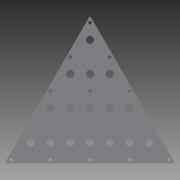
# Autodesk Inventor part: grid16-mask
Saved by Autodesk Inventor 2013 (Build 170138000, 138)
## iProperties
Created: 2013-03-05
Part Number: grid16-mask
Material: Generic
Document SubType Name: Modeling
Designer: Beth Scott
Density: 1 g/cm^3
Author: Beth Scott
Autodesk Inventor part; units mm, degrees
ref_plane "YZ Plane" through (0, 0, 0) normal (1, 0, 0) x (0, 1, 0)
ref_plane "XZ Plane" through (0, 0, 0) normal (0, 1, 0) x (-1, 0, 0)
ref_plane "XY Plane" through (0, 0, 0) normal (0, 0, 1) x (1, 0, 0)
sketch "Triangle 1mm" plane through (0, 0, 0) normal (0, 0, 1) x (1, 0, 0)
  line L0 (0, 0) -> (16.6665, 28.8672) construction
  line L1 (16.6665, 28.8672) -> (33.333, 0) construction
  line L2 (33.333, 0) -> (0, 0) construction
  line L3 (33.333, 0) -> (8.3332, 14.4336) construction
  line L4 (0, 0) -> (24.9997, 14.4336) construction
  line L5 (16.6665, 28.8672) -> (16.6665, 0) construction
  line L6 (0, 14.4336) -> (33.333, 14.4336) construction
  line L7 (0, 19.4336) -> (33.333, 19.4336) construction
  line L8 (0, 9.4336) -> (33.333, 9.4336) construction
  line L9 (16.6665, 19.4336) -> (16.6665, 14.4336) construction
  line L10 (16.6665, 14.4336) -> (16.6665, 9.4336) construction
  circle A0 centre (16.6665, 14.4336) radius 3.5
  point P0 (16.9666, 9.7956)
  dimension "d14" = 33.333
  dimension "d31" = 10
  dimension "d43" = 7
  measures "d14" distance of L1.end L0.start
  measures "d31" distance of L8.start L7.start
  measures "d43" diameter of A0
sketch "Tri16 1mm" plane through (0, 0, 0) normal (0, 0, 1) x (1, 0, 0)
  line L0 (0, 0) -> (16.6665, 28.8672) construction
  line L1 (16.6665, 28.8672) -> (33.333, 0) construction
  line L2 (33.333, 0) -> (0, 0) construction
  line L3 (33.333, 0) -> (8.3333, 14.4336) construction
  line L4 (0, 0) -> (24.9998, 14.4336) construction
  line L5 (16.6665, 28.8672) -> (16.6665, 0) construction
  line L6 (0, 14.4336) -> (33.333, 14.4336) construction
  line L7 (0, 19.4336) -> (33.333, 19.4336) construction
  line L8 (0, 9.4336) -> (33.333, 9.4336) construction
  line L9 (16.6665, 19.4336) -> (16.6665, 14.4336) construction
  line L10 (16.6665, 14.4336) -> (16.6665, 9.4336) construction
  circle A0 centre (16.6665, 14.4336) radius 3.5
  line L11 (33.333, 0) -> (49.9995, 28.8672) construction
  line L12 (49.9995, 28.8672) -> (66.666, 0) construction
  line L13 (66.666, 0) -> (33.333, 0) construction
  line L14 (66.666, 0) -> (41.6663, 14.4336) construction
  line L15 (33.333, 0) -> (58.3328, 14.4336) construction
  line L16 (49.9995, 28.8672) -> (49.9995, 0) construction
  line L17 (33.333, 14.4336) -> (66.666, 14.4336) construction
  line L18 (33.333, 19.4336) -> (66.666, 19.4336) construction
  line L19 (33.333, 9.4336) -> (66.666, 9.4336) construction
  line L20 (49.9995, 19.4336) -> (49.9995, 14.4336) construction
  line L21 (49.9995, 14.4336) -> (49.9995, 9.4336) construction
  circle A1 centre (49.9995, 14.4336) radius 3.5
  line L22 (49.9995, 28.8672) -> (33.333, 0) construction
  line L23 (33.333, 0) -> (16.6665, 28.8672) construction
  line L24 (16.6665, 28.8672) -> (49.9995, 28.8672) construction
  line L25 (16.6665, 28.8672) -> (41.6663, 14.4336) construction
  line L26 (49.9995, 28.8672) -> (24.9998, 14.4336) construction
  line L27 (33.333, 0) -> (33.333, 28.8672) construction
  line L28 (49.9995, 14.4336) -> (16.6665, 14.4336) construction
  line L29 (49.9995, 9.4336) -> (16.6665, 9.4336) construction
  line L30 (49.9995, 19.4336) -> (16.6665, 19.4336) construction
  line L31 (33.333, 9.4336) -> (33.333, 14.4336) construction
  line L32 (33.333, 14.4336) -> (33.333, 19.4336) construction
  circle A2 centre (33.333, 14.4336) radius 3.5
  line L33 (83.3325, 28.8672) -> (66.666, 0) construction
  line L34 (66.666, 0) -> (49.9995, 28.8672) construction
  line L35 (49.9995, 28.8672) -> (83.3325, 28.8672) construction
  line L36 (49.9995, 28.8672) -> (74.9993, 14.4336) construction
  line L37 (83.3325, 28.8672) -> (58.3328, 14.4336) construction
  line L38 (66.666, 0) -> (66.666, 28.8672) construction
  line L39 (83.3325, 14.4336) -> (49.9995, 14.4336) construction
  line L40 (83.3325, 9.4336) -> (49.9995, 9.4336) construction
  line L41 (83.3325, 19.4336) -> (49.9995, 19.4336) construction
  line L42 (66.666, 9.4336) -> (66.666, 14.4336) construction
  line L43 (66.666, 14.4336) -> (66.666, 19.4336) construction
  circle A3 centre (66.666, 14.4336) radius 3.5
  line L44 (66.666, 0) -> (83.3325, 28.8672) construction
  line L45 (83.3325, 28.8672) -> (99.999, 0) construction
  line L46 (99.999, 0) -> (66.666, 0) construction
  line L47 (99.999, 0) -> (74.9993, 14.4336) construction
  line L48 (66.666, 0) -> (91.6658, 14.4336) construction
  line L49 (83.3325, 28.8672) -> (83.3325, 0) construction
  line L50 (66.666, 14.4336) -> (99.999, 14.4336) construction
  line L51 (66.666, 19.4336) -> (99.999, 19.4336) construction
  line L52 (66.666, 9.4336) -> (99.999, 9.4336) construction
  line L53 (83.3325, 19.4336) -> (83.3325, 14.4336) construction
  line L54 (83.3325, 14.4336) -> (83.3325, 9.4336) construction
  circle A4 centre (83.3325, 14.4336) radius 3.5
  line L55 (99.999, 0) -> (116.6655, 28.8672) construction
  line L56 (116.6655, 28.8672) -> (133.332, 0) construction
  line L57 (133.332, 0) -> (99.999, 0) construction
  line L58 (133.332, 0) -> (108.3323, 14.4336) construction
  line L59 (99.999, 0) -> (124.9988, 14.4336) construction
  line L60 (116.6655, 28.8672) -> (116.6655, 0) construction
  line L61 (99.999, 14.4336) -> (133.332, 14.4336) construction
  line L62 (99.999, 19.4336) -> (133.332, 19.4336) construction
  line L63 (99.999, 9.4336) -> (133.332, 9.4336) construction
  line L64 (116.6655, 19.4336) -> (116.6655, 14.4336) construction
  line L65 (116.6655, 14.4336) -> (116.6655, 9.4336) construction
  circle A5 centre (116.6655, 14.4336) radius 3.5
  line L66 (116.6655, 28.8672) -> (99.999, 0) construction
  line L67 (99.999, 0) -> (83.3325, 28.8672) construction
  line L68 (83.3325, 28.8672) -> (116.6655, 28.8672) construction
  line L69 (83.3325, 28.8672) -> (108.3323, 14.4336) construction
  line L70 (116.6655, 28.8672) -> (91.6658, 14.4336) construction
  line L71 (99.999, 0) -> (99.999, 28.8672) construction
  line L72 (116.6655, 14.4336) -> (83.3325, 14.4336) construction
  line L73 (116.6655, 9.4336) -> (83.3325, 9.4336) construction
  line L74 (116.6655, 19.4336) -> (83.3325, 19.4336) construction
  line L75 (99.999, 9.4336) -> (99.999, 14.4336) construction
  line L76 (99.999, 14.4336) -> (99.999, 19.4336) construction
  circle A6 centre (99.999, 14.4336) radius 3.5
  line L77 (16.6665, 28.8672) -> (33.333, 57.7344) construction
  line L78 (33.333, 57.7344) -> (49.9995, 28.8672) construction
  line L79 (49.9995, 28.8672) -> (16.6665, 28.8672) construction
  line L80 (49.9995, 28.8672) -> (24.9998, 43.3008) construction
  line L81 (16.6665, 28.8672) -> (41.6663, 43.3008) construction
  line L82 (33.333, 57.7344) -> (33.333, 28.8672) construction
  line L83 (16.6665, 43.3008) -> (49.9995, 43.3008) construction
  line L84 (16.6665, 48.3008) -> (49.9995, 48.3008) construction
  line L85 (16.6665, 38.3008) -> (49.9995, 38.3008) construction
  line L86 (33.333, 48.3008) -> (33.333, 43.3008) construction
  line L87 (33.333, 43.3008) -> (33.333, 38.3008) construction
  circle A7 centre (33.333, 43.3008) radius 3.5
  line L88 (33.333, 57.7344) -> (49.9995, 86.6017) construction
  line L89 (49.9995, 86.6017) -> (66.666, 57.7344) construction
  line L90 (66.666, 57.7344) -> (33.333, 57.7344) construction
  line L91 (66.666, 57.7344) -> (41.6663, 72.1681) construction
  line L92 (33.333, 57.7344) -> (58.3328, 72.1681) construction
  line L93 (49.9995, 86.6017) -> (49.9995, 57.7344) construction
  line L94 (33.333, 72.1681) -> (66.666, 72.1681) construction
  line L95 (33.333, 77.1681) -> (66.666, 77.1681) construction
  line L96 (33.333, 67.1681) -> (66.666, 67.1681) construction
  line L97 (49.9995, 77.1681) -> (49.9995, 72.1681) construction
  line L98 (49.9995, 72.1681) -> (49.9995, 67.1681) construction
  circle A8 centre (49.9995, 72.1681) radius 3.5
  line L99 (49.9995, 86.6017) -> (66.666, 115.4689) construction
  line L100 (66.666, 115.4689) -> (83.3325, 86.6017) construction
  line L101 (83.3325, 86.6017) -> (49.9995, 86.6017) construction
  line L102 (83.3325, 86.6017) -> (58.3328, 101.0353) construction
  line L103 (49.9995, 86.6017) -> (74.9993, 101.0353) construction
  line L104 (66.666, 115.4689) -> (66.666, 86.6017) construction
  line L105 (49.9995, 101.0353) -> (83.3325, 101.0353) construction
  line L106 (49.9995, 106.0353) -> (83.3325, 106.0353) construction
  line L107 (49.9995, 96.0353) -> (83.3325, 96.0353) construction
  line L108 (66.666, 106.0353) -> (66.666, 101.0353) construction
  line L109 (66.666, 101.0353) -> (66.666, 96.0353) construction
  circle A9 centre (66.666, 101.0353) radius 3.5
  line L110 (66.666, 57.7344) -> (49.9995, 28.8672) construction
  line L111 (49.9995, 28.8672) -> (33.333, 57.7344) construction
  line L112 (33.333, 57.7344) -> (66.666, 57.7344) construction
  line L113 (33.333, 57.7344) -> (58.3328, 43.3008) construction
  line L114 (66.666, 57.7344) -> (41.6663, 43.3008) construction
  line L115 (49.9995, 28.8672) -> (49.9995, 57.7344) construction
  line L116 (66.666, 43.3008) -> (33.333, 43.3008) construction
  line L117 (66.666, 38.3008) -> (33.333, 38.3008) construction
  line L118 (66.666, 48.3008) -> (33.333, 48.3008) construction
  line L119 (49.9995, 38.3008) -> (49.9995, 43.3008) construction
  line L120 (49.9995, 43.3008) -> (49.9995, 48.3008) construction
  circle A10 centre (49.9995, 43.3008) radius 3.5
  line L121 (83.3325, 86.6017) -> (66.666, 57.7344) construction
  line L122 (66.666, 57.7344) -> (49.9995, 86.6017) construction
  line L123 (49.9995, 86.6017) -> (83.3325, 86.6017) construction
  line L124 (49.9995, 86.6017) -> (74.9993, 72.1681) construction
  line L125 (83.3325, 86.6017) -> (58.3328, 72.1681) construction
  line L126 (66.666, 57.7344) -> (66.666, 86.6017) construction
  line L127 (83.3325, 72.1681) -> (49.9995, 72.1681) construction
  line L128 (83.3325, 67.1681) -> (49.9995, 67.1681) construction
  line L129 (83.3325, 77.1681) -> (49.9995, 77.1681) construction
  line L130 (66.666, 67.1681) -> (66.666, 72.1681) construction
  line L131 (66.666, 72.1681) -> (66.666, 77.1681) construction
  circle A11 centre (66.666, 72.1681) radius 3.5
  line L132 (66.666, 57.7344) -> (83.3325, 86.6017) construction
  line L133 (83.3325, 86.6017) -> (99.999, 57.7344) construction
  line L134 (99.999, 57.7344) -> (66.666, 57.7344) construction
  line L135 (99.999, 57.7344) -> (74.9993, 72.1681) construction
  line L136 (66.666, 57.7344) -> (91.6658, 72.1681) construction
  line L137 (83.3325, 86.6017) -> (83.3325, 57.7344) construction
  line L138 (66.666, 72.1681) -> (99.999, 72.1681) construction
  line L139 (66.666, 77.1681) -> (99.999, 77.1681) construction
  line L140 (66.666, 67.1681) -> (99.999, 67.1681) construction
  line L141 (83.3325, 77.1681) -> (83.3325, 72.1681) construction
  line L142 (83.3325, 72.1681) -> (83.3325, 67.1681) construction
  circle A12 centre (83.3325, 72.1681) radius 3.5
  line L143 (49.9995, 28.8672) -> (66.666, 57.7344) construction
  line L144 (66.666, 57.7344) -> (83.3325, 28.8672) construction
  line L145 (83.3325, 28.8672) -> (49.9995, 28.8672) construction
  line L146 (83.3325, 28.8672) -> (58.3328, 43.3008) construction
  line L147 (49.9995, 28.8672) -> (74.9993, 43.3008) construction
  line L148 (66.666, 57.7344) -> (66.666, 28.8672) construction
  line L149 (49.9995, 43.3008) -> (83.3325, 43.3008) construction
  line L150 (49.9995, 48.3008) -> (83.3325, 48.3008) construction
  line L151 (49.9995, 38.3008) -> (83.3325, 38.3008) construction
  line L152 (66.666, 48.3008) -> (66.666, 43.3008) construction
  line L153 (66.666, 43.3008) -> (66.666, 38.3008) construction
  circle A13 centre (66.666, 43.3008) radius 3.5
  line L154 (83.3325, 28.8672) -> (99.999, 57.7344) construction
  line L155 (99.999, 57.7344) -> (116.6655, 28.8672) construction
  line L156 (116.6655, 28.8672) -> (83.3325, 28.8672) construction
  line L157 (116.6655, 28.8672) -> (91.6658, 43.3008) construction
  line L158 (83.3325, 28.8672) -> (108.3323, 43.3008) construction
  line L159 (99.999, 57.7344) -> (99.999, 28.8672) construction
  line L160 (83.3325, 43.3008) -> (116.6655, 43.3008) construction
  line L161 (83.3325, 48.3008) -> (116.6655, 48.3008) construction
  line L162 (83.3325, 38.3008) -> (116.6655, 38.3008) construction
  line L163 (99.999, 48.3008) -> (99.999, 43.3008) construction
  line L164 (99.999, 43.3008) -> (99.999, 38.3008) construction
  circle A14 centre (99.999, 43.3008) radius 3.5
  line L165 (99.999, 57.7344) -> (83.3325, 28.8672) construction
  line L166 (83.3325, 28.8672) -> (66.666, 57.7344) construction
  line L167 (66.666, 57.7344) -> (99.999, 57.7344) construction
  line L168 (66.666, 57.7344) -> (91.6658, 43.3008) construction
  line L169 (99.999, 57.7344) -> (74.9993, 43.3008) construction
  line L170 (83.3325, 28.8672) -> (83.3325, 57.7344) construction
  line L171 (99.999, 43.3008) -> (66.666, 43.3008) construction
  line L172 (99.999, 38.3008) -> (66.666, 38.3008) construction
  line L173 (99.999, 48.3008) -> (66.666, 48.3008) construction
  line L174 (83.3325, 38.3008) -> (83.3325, 43.3008) construction
  line L175 (83.3325, 43.3008) -> (83.3325, 48.3008) construction
  circle A15 centre (83.3325, 43.3008) radius 3.5
  point P0 (66.741, 38.5329)
sketch "Top Plate" plane through (0, 0, 0) normal (0, 1, 0) x (-1, 0, 0)
  line L0 (-4.3301, -1.5) -> (65.8, 119.9689)
  line L1 (67.532, 119.9689) -> (137.6621, -1.5)
  line L2 (-3.4641, -3) -> (136.7961, -3)
  circle A0 centre (33.333, 0) radius 1.5
  circle A1 centre (0, 0) radius 1.5
  circle A2 centre (16.6665, 28.8672) radius 1.5
  circle A3 centre (33.333, 57.7344) radius 1.5
  circle A4 centre (49.9995, 28.8672) radius 1.5
  circle A5 centre (66.666, 0) radius 1.5
  circle A6 centre (99.999, 0) radius 1.5
  circle A7 centre (133.332, 0) radius 1.5
  circle A8 centre (116.6655, 28.8672) radius 1.5
  circle A9 centre (99.999, 57.7344) radius 1.5
  circle A10 centre (83.3325, 28.8672) radius 1.5
  circle A11 centre (66.666, 57.7344) radius 1.5
  circle A12 centre (83.3325, 86.6017) radius 1.5
  circle A13 centre (49.9995, 86.6017) radius 1.5
  circle A14 centre (66.666, 115.4689) radius 1.5
  arc A15 (67.532, 119.9689) -> (65.8, 119.9689) centre (66.666, 119.4689) ccw
  arc A16 (136.7961, -3) -> (137.6621, -1.5) centre (136.7961, -2) ccw
  arc A17 (-4.3301, -1.5) -> (-3.4641, -3) centre (-3.4641, -2) ccw
  line L3 (0, 0) -> (-14.4563, -8.3464) construction
  line L4 (133.332, 0) -> (144.2364, -6.2956) construction
  line L5 (27.8865, 48.3008) -> (27.8865, 48.3008)
  line L6 (108.6655, 28.8672) -> (113.6655, 28.8672) construction
  line L7 (98.999, 38.3008) -> (99.999, 38.3008)
  line L8 (0, 0) -> (16.6665, 28.8672) construction
  line L9 (16.6665, 28.8672) -> (33.333, 0) construction
  line L10 (33.333, 0) -> (0, 0) construction
  line L11 (33.333, 0) -> (8.3333, 14.4336) construction
  line L12 (0, 0) -> (24.9998, 14.4336) construction
  line L13 (16.6665, 28.8672) -> (16.6665, 0) construction
  line L14 (0, 14.4336) -> (33.333, 14.4336) construction
  line L15 (0, 19.4336) -> (33.333, 19.4336) construction
  line L16 (0, 9.4336) -> (33.333, 9.4336) construction
  line L17 (16.6665, 19.4336) -> (16.6665, 14.4336) construction
  line L18 (16.6665, 14.4336) -> (16.6665, 9.4336) construction
  circle A18 centre (16.6665, 14.4336) radius 3.5
  line L19 (33.333, 0) -> (49.9995, 28.8672) construction
  line L20 (49.9995, 28.8672) -> (66.666, 0) construction
  line L21 (66.666, 0) -> (33.333, 0) construction
  line L22 (66.666, 0) -> (41.6663, 14.4336) construction
  line L23 (33.333, 0) -> (58.3328, 14.4336) construction
  line L24 (49.9995, 28.8672) -> (49.9995, 0) construction
  line L25 (33.333, 14.4336) -> (66.666, 14.4336) construction
  line L26 (33.333, 19.4336) -> (66.666, 19.4336) construction
  line L27 (33.333, 9.4336) -> (66.666, 9.4336) construction
  line L28 (49.9995, 19.4336) -> (49.9995, 14.4336) construction
  line L29 (49.9995, 14.4336) -> (49.9995, 9.4336) construction
  circle A19 centre (49.9995, 14.4336) radius 3.5
  line L30 (49.9995, 28.8672) -> (33.333, 0) construction
  line L31 (33.333, 0) -> (16.6665, 28.8672) construction
  line L32 (16.6665, 28.8672) -> (49.9995, 28.8672) construction
  line L33 (16.6665, 28.8672) -> (41.6663, 14.4336) construction
  line L34 (49.9995, 28.8672) -> (24.9998, 14.4336) construction
  line L35 (33.333, 0) -> (33.333, 28.8672) construction
  line L36 (49.9995, 14.4336) -> (16.6665, 14.4336) construction
  line L37 (49.9995, 9.4336) -> (16.6665, 9.4336) construction
  line L38 (49.9995, 19.4336) -> (16.6665, 19.4336) construction
  line L39 (33.333, 9.4336) -> (33.333, 14.4336) construction
  line L40 (33.333, 14.4336) -> (33.333, 19.4336) construction
  circle A20 centre (33.333, 14.4336) radius 3.5
  line L41 (83.3325, 28.8672) -> (66.666, 0) construction
  line L42 (66.666, 0) -> (49.9995, 28.8672) construction
  line L43 (49.9995, 28.8672) -> (83.3325, 28.8672) construction
  line L44 (49.9995, 28.8672) -> (74.9993, 14.4336) construction
  line L45 (83.3325, 28.8672) -> (58.3328, 14.4336) construction
  line L46 (66.666, 0) -> (66.666, 28.8672) construction
  line L47 (83.3325, 14.4336) -> (49.9995, 14.4336) construction
  line L48 (83.3325, 9.4336) -> (49.9995, 9.4336) construction
  line L49 (83.3325, 19.4336) -> (49.9995, 19.4336) construction
  line L50 (66.666, 9.4336) -> (66.666, 14.4336) construction
  line L51 (66.666, 14.4336) -> (66.666, 19.4336) construction
  circle A21 centre (66.666, 14.4336) radius 3.5
  line L52 (66.666, 0) -> (83.3325, 28.8672) construction
  line L53 (83.3325, 28.8672) -> (99.999, 0) construction
  line L54 (99.999, 0) -> (66.666, 0) construction
  line L55 (99.999, 0) -> (74.9993, 14.4336) construction
  line L56 (66.666, 0) -> (91.6658, 14.4336) construction
  line L57 (83.3325, 28.8672) -> (83.3325, 0) construction
  line L58 (66.666, 14.4336) -> (99.999, 14.4336) construction
  line L59 (66.666, 19.4336) -> (99.999, 19.4336) construction
  line L60 (66.666, 9.4336) -> (99.999, 9.4336) construction
  line L61 (83.3325, 19.4336) -> (83.3325, 14.4336) construction
  line L62 (83.3325, 14.4336) -> (83.3325, 9.4336) construction
  circle A22 centre (83.3325, 14.4336) radius 3.5
  line L63 (99.999, 0) -> (116.6655, 28.8672) construction
  line L64 (116.6655, 28.8672) -> (133.332, 0) construction
  line L65 (133.332, 0) -> (99.999, 0) construction
  line L66 (133.332, 0) -> (108.3323, 14.4336) construction
  line L67 (99.999, 0) -> (124.9988, 14.4336) construction
  line L68 (116.6655, 28.8672) -> (116.6655, 0) construction
  line L69 (99.999, 14.4336) -> (133.332, 14.4336) construction
  line L70 (99.999, 19.4336) -> (133.332, 19.4336) construction
  line L71 (99.999, 9.4336) -> (133.332, 9.4336) construction
  line L72 (116.6655, 19.4336) -> (116.6655, 14.4336) construction
  line L73 (116.6655, 14.4336) -> (116.6655, 9.4336) construction
  circle A23 centre (116.6655, 14.4336) radius 3.5
  line L74 (116.6655, 28.8672) -> (99.999, 0) construction
  line L75 (99.999, 0) -> (83.3325, 28.8672) construction
  line L76 (83.3325, 28.8672) -> (116.6655, 28.8672) construction
  line L77 (83.3325, 28.8672) -> (108.3323, 14.4336) construction
  line L78 (116.6655, 28.8672) -> (91.6658, 14.4336) construction
  line L79 (99.999, 0) -> (99.999, 28.8672) construction
  line L80 (116.6655, 14.4336) -> (83.3325, 14.4336) construction
  line L81 (116.6655, 9.4336) -> (83.3325, 9.4336) construction
  line L82 (116.6655, 19.4336) -> (83.3325, 19.4336) construction
  line L83 (99.999, 9.4336) -> (99.999, 14.4336) construction
  line L84 (99.999, 14.4336) -> (99.999, 19.4336) construction
  circle A24 centre (99.999, 14.4336) radius 3.5
  line L85 (16.6665, 28.8672) -> (33.333, 57.7344) construction
  line L86 (33.333, 57.7344) -> (49.9995, 28.8672) construction
  line L87 (49.9995, 28.8672) -> (16.6665, 28.8672) construction
  line L88 (49.9995, 28.8672) -> (24.9998, 43.3008) construction
  line L89 (16.6665, 28.8672) -> (41.6663, 43.3008) construction
  line L90 (33.333, 57.7344) -> (33.333, 28.8672) construction
  line L91 (16.6665, 43.3008) -> (49.9995, 43.3008) construction
  line L92 (16.6665, 48.3008) -> (49.9995, 48.3008) construction
  line L93 (16.6665, 38.3008) -> (49.9995, 38.3008) construction
  line L94 (33.333, 48.3008) -> (33.333, 43.3008) construction
  line L95 (33.333, 43.3008) -> (33.333, 38.3008) construction
  circle A25 centre (33.333, 43.3008) radius 3.5
  line L96 (33.333, 57.7344) -> (49.9995, 86.6017) construction
  line L97 (49.9995, 86.6017) -> (66.666, 57.7344) construction
  line L98 (66.666, 57.7344) -> (33.333, 57.7344) construction
  line L99 (66.666, 57.7344) -> (41.6663, 72.1681) construction
  line L100 (33.333, 57.7344) -> (58.3328, 72.1681) construction
  line L101 (49.9995, 86.6017) -> (49.9995, 57.7344) construction
  line L102 (33.333, 72.1681) -> (66.666, 72.1681) construction
  line L103 (33.333, 77.1681) -> (66.666, 77.1681) construction
  line L104 (33.333, 67.1681) -> (66.666, 67.1681) construction
  line L105 (49.9995, 77.1681) -> (49.9995, 72.1681) construction
  line L106 (49.9995, 72.1681) -> (49.9995, 67.1681) construction
  circle A26 centre (49.9995, 72.1681) radius 3.5
  line L107 (49.9995, 86.6017) -> (66.666, 115.4689) construction
  line L108 (66.666, 115.4689) -> (83.3325, 86.6017) construction
  line L109 (83.3325, 86.6017) -> (49.9995, 86.6017) construction
  line L110 (83.3325, 86.6017) -> (58.3328, 101.0353) construction
  line L111 (49.9995, 86.6017) -> (74.9993, 101.0353) construction
  line L112 (66.666, 115.4689) -> (66.666, 86.6017) construction
  line L113 (49.9995, 101.0353) -> (83.3325, 101.0353) construction
  line L114 (49.9995, 106.0353) -> (83.3325, 106.0353) construction
  line L115 (49.9995, 96.0353) -> (83.3325, 96.0353) construction
  line L116 (66.666, 106.0353) -> (66.666, 101.0353) construction
  line L117 (66.666, 101.0353) -> (66.666, 96.0353) construction
  circle A27 centre (66.666, 101.0353) radius 3.5
  line L118 (66.666, 57.7344) -> (49.9995, 28.8672) construction
  line L119 (49.9995, 28.8672) -> (33.333, 57.7344) construction
  line L120 (33.333, 57.7344) -> (66.666, 57.7344) construction
  line L121 (33.333, 57.7344) -> (58.3328, 43.3008) construction
  line L122 (66.666, 57.7344) -> (41.6663, 43.3008) construction
  line L123 (49.9995, 28.8672) -> (49.9995, 57.7344) construction
  line L124 (66.666, 43.3008) -> (33.333, 43.3008) construction
  line L125 (66.666, 38.3008) -> (33.333, 38.3008) construction
  line L126 (66.666, 48.3008) -> (33.333, 48.3008) construction
  line L127 (49.9995, 38.3008) -> (49.9995, 43.3008) construction
  line L128 (49.9995, 43.3008) -> (49.9995, 48.3008) construction
  circle A28 centre (49.9995, 43.3008) radius 3.5
  line L129 (83.3325, 86.6017) -> (66.666, 57.7344) construction
  line L130 (66.666, 57.7344) -> (49.9995, 86.6017) construction
  line L131 (49.9995, 86.6017) -> (83.3325, 86.6017) construction
  line L132 (49.9995, 86.6017) -> (74.9993, 72.1681) construction
  line L133 (83.3325, 86.6017) -> (58.3328, 72.1681) construction
  line L134 (66.666, 57.7344) -> (66.666, 86.6017) construction
  line L135 (83.3325, 72.1681) -> (49.9995, 72.1681) construction
  line L136 (83.3325, 67.1681) -> (49.9995, 67.1681) construction
  line L137 (83.3325, 77.1681) -> (49.9995, 77.1681) construction
  line L138 (66.666, 67.1681) -> (66.666, 72.1681) construction
  line L139 (66.666, 72.1681) -> (66.666, 77.1681) construction
  circle A29 centre (66.666, 72.1681) radius 3.5
  line L140 (66.666, 57.7344) -> (83.3325, 86.6017) construction
  line L141 (83.3325, 86.6017) -> (99.999, 57.7344) construction
  line L142 (99.999, 57.7344) -> (66.666, 57.7344) construction
  line L143 (99.999, 57.7344) -> (74.9993, 72.1681) construction
  line L144 (66.666, 57.7344) -> (91.6658, 72.1681) construction
  line L145 (83.3325, 86.6017) -> (83.3325, 57.7344) construction
  line L146 (66.666, 72.1681) -> (99.999, 72.1681) construction
  line L147 (66.666, 77.1681) -> (99.999, 77.1681) construction
  line L148 (66.666, 67.1681) -> (99.999, 67.1681) construction
  line L149 (83.3325, 77.1681) -> (83.3325, 72.1681) construction
  line L150 (83.3325, 72.1681) -> (83.3325, 67.1681) construction
  circle A30 centre (83.3325, 72.1681) radius 3.5
  line L151 (49.9995, 28.8672) -> (66.666, 57.7344) construction
  line L152 (66.666, 57.7344) -> (83.3325, 28.8672) construction
  line L153 (83.3325, 28.8672) -> (49.9995, 28.8672) construction
  line L154 (83.3325, 28.8672) -> (58.3328, 43.3008) construction
  line L155 (49.9995, 28.8672) -> (74.9993, 43.3008) construction
  line L156 (66.666, 57.7344) -> (66.666, 28.8672) construction
  line L157 (49.9995, 43.3008) -> (83.3325, 43.3008) construction
  line L158 (49.9995, 48.3008) -> (83.3325, 48.3008) construction
  line L159 (49.9995, 38.3008) -> (83.3325, 38.3008) construction
  line L160 (66.666, 48.3008) -> (66.666, 43.3008) construction
  line L161 (66.666, 43.3008) -> (66.666, 38.3008) construction
  circle A31 centre (66.666, 43.3008) radius 3.5
  line L162 (83.3325, 28.8672) -> (99.999, 57.7344) construction
  line L163 (99.999, 57.7344) -> (116.6655, 28.8672) construction
  line L164 (116.6655, 28.8672) -> (83.3325, 28.8672) construction
  line L165 (116.6655, 28.8672) -> (91.6658, 43.3008) construction
  line L166 (83.3325, 28.8672) -> (108.3323, 43.3008) construction
  line L167 (99.999, 57.7344) -> (99.999, 28.8672) construction
  line L168 (83.3325, 43.3008) -> (116.6655, 43.3008) construction
  line L169 (83.3325, 48.3008) -> (116.6655, 48.3008) construction
  line L170 (83.3325, 38.3008) -> (116.6655, 38.3008) construction
  line L171 (99.999, 48.3008) -> (99.999, 43.3008) construction
  line L172 (99.999, 43.3008) -> (99.999, 38.3008) construction
  circle A32 centre (99.999, 43.3008) radius 3.5
  line L173 (99.999, 57.7344) -> (83.3325, 28.8672) construction
  line L174 (83.3325, 28.8672) -> (66.666, 57.7344) construction
  line L175 (66.666, 57.7344) -> (99.999, 57.7344) construction
  line L176 (66.666, 57.7344) -> (91.6658, 43.3008) construction
  line L177 (99.999, 57.7344) -> (74.9993, 43.3008) construction
  line L178 (83.3325, 28.8672) -> (83.3325, 57.7344) construction
  line L179 (99.999, 43.3008) -> (66.666, 43.3008) construction
  line L180 (99.999, 38.3008) -> (66.666, 38.3008) construction
  line L181 (99.999, 48.3008) -> (66.666, 48.3008) construction
  line L182 (83.3325, 38.3008) -> (83.3325, 43.3008) construction
  line L183 (83.3325, 43.3008) -> (83.3325, 48.3008) construction
  circle A33 centre (83.3325, 43.3008) radius 3.5
  dimension "d25" = 3
  dimension "d35" = 3
  dimension "d36" = 1
  constraints: 18 centre point, 16 end point, 16 equal radius, 6 point on circle, 6 tangent, 3 horizontal, 2 point on line, 26 other
  measures "d25" diameter of A0
  measures "d35" distance from line of L2 A6.centre
  measures "d36" radius of A16
extrude "Extrusion3" add sketch "Top Plate" along normal blind 6
body "Solid3"
